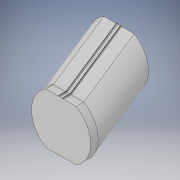
# Autodesk Inventor part: ramp bottom connect
Saved by Autodesk Inventor 2017 (Build 210142000, 142)
## iProperties
Created: 2018-03-06
Part Number: ramp bottom connect
Material: Generic
Document SubType Name: Modeling
Designer: braxtonwright
Density: 1 g/cm^3
Appearance: Default
Author: braxtonwright
Autodesk Inventor part; units mm, degrees
ref_plane "YZ Plane" through (0, 0, 0) normal (1, 0, 0) x (0, 1, 0)
ref_plane "XZ Plane" through (0, 0, 0) normal (0, 1, 0) x (-1, 0, 0)
ref_plane "XY Plane" through (0, 0, 0) normal (0, 0, 1) x (1, 0, 0)
sketch "Sketch1" plane through (0, 0, 0) normal (0, 0, 1) x (1, 0, 0)
  line L0 (6.35, 87.8623) -> (6.35, 86.6385)
  line L1 (7.4083, 87.8623) -> (6.35, 87.8623)
  arc A0 (4.1034, 84.6667) -> (6.35, 86.6385) centre (4.1034, 86.9324) ccw
  line L2 (6.3485, 84.6873) -> (3.1735, 87.8623) construction
  arc A1 (6.35, 87.8623) -> (3.1736, 84.6667) centre (6.3485, 84.6873) ccw construction
  line L3 (0, 84.6667) -> (0, 87.8623) construction
  line L4 (6.35, 87.8623) -> (0, 87.8623) construction
  line L5 (-6.35, 87.8623) -> (0, 87.8623) construction
  arc A2 (-3.1736, 84.6667) -> (-6.35, 87.8623) centre (-6.3485, 84.6873) ccw construction
  line L6 (-6.35, 87.8623) -> (-6.35, 86.6385)
  arc A3 (-6.35, 86.6385) -> (-4.1034, 84.6667) centre (-4.1034, 86.9324) ccw
  line L7 (-7.4083, 87.8623) -> (-7.4083, 86.2542)
  line L8 (-6.35, 87.8623) -> (-7.4083, 87.8623)
  arc A4 (-8.9958, 84.6667) -> (-7.4083, 86.2542) centre (-8.9958, 86.2542) ccw
  line L9 (-6.3485, 84.6873) -> (-3.1735, 87.8623) construction
  line L10 (4.1034, 84.6667) -> (0, 84.6667)
  line L11 (-8.9958, 84.6667) -> (-50.8, 84.6667)
  line L12 (8.9958, 84.6667) -> (50.8, 84.6667)
  arc A5 (-50.8, 84.6667) -> (-50.8, -84.6667) centre (0, 0) ccw
  line L13 (-50.8, -84.6667) -> (50.8, -84.6667)
  arc A6 (50.8, -84.6667) -> (50.8, 84.6667) centre (0, 0) ccw
  line L14 (-4.1034, 84.6667) -> (0, 84.6667)
  line L15 (-8.9958, 84.6667) -> (8.9958, 84.6667) construction
  arc A7 (7.4083, 86.2542) -> (8.9958, 84.6667) centre (8.9958, 86.2542) ccw
  line L16 (7.4083, 87.8623) -> (7.4083, 86.2542)
  dimension "d30" = 0
  dimension "d110" = 101.6
  dimension "d111" = 14.8167
  dimension "d112" = 98.7374
  dimension "d113" = 98.7374
  dimension "d114" = 43.3917
  dimension "d115" = 1.5875
  dimension "d116" = 1.5875
  dimension "d117" = 41.8042
  dimension "d118" = 6.35
  dimension "d119" = 3.175
  dimension "d120" = 2.2657
  dimension "d121" = 2.2466
  dimension "d122" = 45
  dimension "d123" = 84.6667
  constraints: 34 end point, 19 point on circle, 8 centre point, 7 symmetric about line, 6 point on line, 5 collinear, 4 perpendicular, 3 coincident, 3 equal length, 2 tangent, 1 equal radius, 1 horizontal, 1 parallel, 3 other
  measures "d110" distance of L11.end L12.end
  measures "d111" distance of L8.end L1.start
  measures "d112" radius of A5
  measures "d113" radius of A6
  measures "d114" distance from line of L11.end L7
  measures "d115" distance from line of L12.start L16
  measures "d116" radius of A7
  measures "d117" distance of L12.start L12.end
  measures "d118" distance of L3.end L6.start
  measures "d119" distance of L6.start L9.start
  measures "d120" radius of A3
  measures "d121" horizontal distance of L14.start L6.end
  measures "d122" angle of L5 L9
  measures "d123" distance from line of L13 point (0, 0)
ref_plane "Work Plane2" through (0, 0, 203.2) normal (0, 0, 1) x (1, 0, 0)
sketch "Sketch6" plane through (0, 0, 0) normal (1, 0, 0) x (0, 1, 0)
  line L0 (-83.4784, 0) -> (-197.1064, 168.4604)
  line L1 (-83.4784, 0) -> (85.0362, 0) construction
  point P0 (0, 0)
  dimension "d28" = 203.2
  dimension "d62" = 124
  constraints: 4 end point, 1 horizontal
  measures "d28" distance of L0.start L0.end
  measures "d62" angle of L1 L0
sweep "ramp" add profiles "Sketch1" path "Sketch6"
sketch "Sketch7" plane through (0, -116.5507, 168.4604) normal (0, 0, 1) x (1, 0, 0)
  line L0 (-50.8, -81.7439) -> (50.8, -81.7439)
  arc A0 (-50.8, 87.5894) -> (-50.8, -81.7439) centre (0, 2.9227) ccw
  arc A1 (50.8, -81.7439) -> (50.8, 87.5894) centre (0, 2.9227) ccw
  line L1 (0, 84.67) -> (0, 90.785) construction
  line L2 (-7.4083, 90.785) -> (-7.4083, 89.1769)
  line L3 (7.4083, 90.785) -> (7.4083, 89.1769)
  line L4 (8.9958, 87.5894) -> (50.8, 87.5894)
  line L5 (-8.9958, 87.5894) -> (8.9958, 87.5894) construction
  arc A2 (7.4083, 89.1769) -> (8.9958, 87.5894) centre (8.9958, 89.1769) ccw
  arc A3 (-8.9958, 87.5894) -> (-7.4083, 89.1769) centre (-8.9958, 89.1769) ccw
  line L6 (-8.9958, 87.5894) -> (-50.8, 87.5894)
  line L7 (0, 87.5894) -> (0, 90.785) construction
  line L8 (6.35, 90.785) -> (0, 90.785) construction
  line L9 (6.3485, 87.61) -> (3.1735, 90.785) construction
  arc A4 (6.35, 90.785) -> (3.1736, 87.5894) centre (6.3485, 87.61) ccw construction
  arc A5 (4.1034, 87.5894) -> (6.35, 89.5612) centre (4.1034, 89.8551) ccw
  line L10 (6.35, 90.785) -> (6.35, 89.5612)
  line L11 (-4.1034, 87.5894) -> (0, 87.5894)
  line L12 (-6.3485, 87.61) -> (-3.1735, 90.785) construction
  line L13 (-6.35, 90.785) -> (-6.35, 89.5612)
  line L14 (-6.35, 90.785) -> (0, 90.785) construction
  arc A6 (-6.35, 89.5612) -> (-4.1034, 87.5894) centre (-4.1034, 89.8551) ccw
  arc A7 (-3.1736, 87.5894) -> (-6.35, 90.785) centre (-6.3485, 87.61) ccw construction
  line L15 (4.1034, 87.5894) -> (0, 87.5894)
  line L16 (7.4083, 90.785) -> (6.35, 90.785)
  line L17 (-6.35, 90.785) -> (-7.4083, 90.785)
  arc A8 (-50.8, 87.5894) -> (-50.8, -81.7439) centre (0, 2.9227) ccw projected
  dimension "d125" = 101.6
  dimension "d126" = 14.8167
  dimension "d127" = 98.7374
  dimension "d128" = 98.7374
  dimension "d129" = 43.3917
  dimension "d130" = 1.5875
  dimension "d131" = 1.5875
  dimension "d132" = 41.8042
  dimension "d133" = 6.35
  dimension "d134" = 3.175
  dimension "d135" = 2.2657
  dimension "d136" = 2.2466
  dimension "d137" = 45
  dimension "d138" = 84.6667
  constraints: 36 end point, 19 point on circle, 10 symmetric about line, 8 centre point, 6 point on line, 4 coincident, 4 collinear, 4 perpendicular, 2 horizontal, 2 tangent, 1 parallel, 1 vertical, 3 other
  measures "d125" distance of L6.end L4.end
  measures "d126" distance of L2.start L3.start
  measures "d127" radius of A0
  measures "d128" radius of A1
  measures "d129" distance from line of L6.end L2
  measures "d130" distance from line of L4.start L3
  measures "d131" radius of A2
  measures "d132" distance of L4.start L4.end
  measures "d133" distance of L1.end L14.start
  measures "d134" distance of L14.start L12.start
  measures "d135" radius of A6
  measures "d136" horizontal distance of L11.start L13.end
  measures "d137" angle of L14 L12
  measures "d138" distance from line of L0 point (0, 2.923)
extrude "connection bottom" add sketch "Sketch7" along normal blind 25.4
equation "\"d113\" = d112"
equation "\"d115\" = 0.5 * d124"
equation "\"d128\" = d127"
equation "\"d130\" = 0.5 * d139"
equation "\"d124\" = 3.175"
equation "\"d139\" = 3.175"
body "Solid1"
